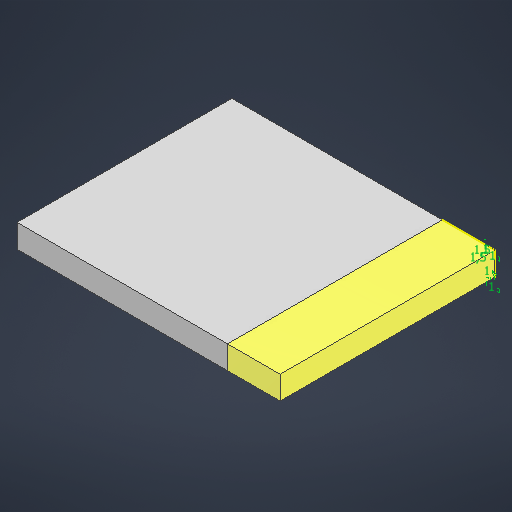
# Autodesk Inventor part: bateria
Saved by Autodesk Inventor 2026.2 (Build 302298000, 298)
## iProperties
Created: 2025-06-11
Part Number: bateria
Material: Generic
Document SubType Name: Modeling
Designer: cdavi
Density: 1 g/cm^3
Appearance: Default
Mass: 15.5961 g
Surface Area: 75.925 cm^2
Volume: 15.5961 cm^3
Author: cdavi
Autodesk Inventor part; units mm, degrees
ref_plane "YZ Plane" through (0, 0, 0) normal (1, 0, 0) x (0, 1, 0)
ref_plane "XZ Plane" through (0, 0, 0) normal (0, 1, 0) x (-1, 0, 0)
ref_plane "XY Plane" through (0, 0, 0) normal (0, 0, 1) x (1, 0, 0)
sketch "Sketch1" plane through (0, 0, 0) normal (0, 1, 0) x (-1, 0, 0)
  line L0 (0, 0) -> (60, 0)
  line L1 (60, 0) -> (60, -49)
  line L2 (60, -49) -> (0, -49)
  line L3 (0, -49) -> (0, 0)
  dimension "d0" = 60
  dimension "d1" = 49
  constraints: 8 end point, 2 parallel, 1 horizontal, 1 perpendicular
  measures "d0" distance of L1.end L2.end
  measures "d1" distance of L0.end L1.end
extrude "Extrusion1" add sketch "Sketch1" along normal blind 5.3
sketch "Sketch2" plane through (0, 5.3, 0) normal (0, 1, 0) x (1, 0, 0)
  line L0 (-60, 0) -> (0, 0) projected
  line L1 (-12, 0) -> (-12, 49)
  line L2 (0, 49) -> (-60, 49) projected
  line L3 (0, 0) -> (0, 49) projected
  dimension "d4" = 12
  constraints: 2 end point, 2 point on line, 1 vertical
  measures "d4" distance between parallel lines of L3 L1
split body "Split1" sketch "Sketch2" result two bodies curves L1 first body at (-44, 0.5, -32.6667)
sketch "Sketch3" plane through (0, 0, -49) normal (0, 0, -1) x (-1, 0, 0)
  circle A0 centre (1, 4.3) radius 0.75
  circle A1 centre (1, 1) radius 0.75
  line L0 (0, 0) -> (0, 5.3) projected
  line L1 (0, 5.3) -> (12, 5.3) projected
  line L2 (0, 0) -> (12, 0) projected
  dimension "d5" = 1
  dimension "d6" = 1
  dimension "d7" = 1.5
  dimension "d8" = 1.5
  dimension "d9" = 1
  dimension "d10" = 1
  constraints: 2 centre point
  measures "d5" distance from line of L0 A0.centre
  measures "d6" distance from line of L0 A1.centre
  measures "d7" diameter of A1
  measures "d8" diameter of A0
  measures "d9" distance from line of L1 A0.centre
  measures "d10" distance from line of L2 A1.centre
body "Solid2"
body "Solid3"
